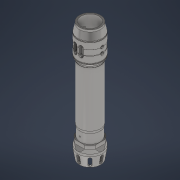
# Autodesk Inventor part: TestPiece1
Saved by Autodesk Inventor 2022 (Build 260153000, 153)
## iProperties
Created: 2024-05-07
Part Number: TestPiece1
Material: Generic
Document SubType Name: Modeling
Designer: jo_ki
Density: 1 g/cm^3
Appearance: Steel - Polished
Author: jo_ki
Autodesk Inventor part; units mm, degrees
sketch "Sketch3" plane through (0, 0, 0) normal (0, 0, 1) x (1, 0, 0)
  line L0 (0, 0) -> (18.25, 0)
  line L1 (18.25, 0) -> (18.25, 106.5)
  line L2 (18.25, 106.5) -> (0, 106.5)
  line L3 (0, 106.5) -> (0, 0)
  line L4 (18.25, 4) -> (18.75, 4)
  line L5 (18.75, 4) -> (18.75, 102.5)
  line L6 (18.75, 102.5) -> (18.25, 102.5)
  line L7 (18.25, 102.5) -> (18.25, 4)
  line L8 (0, -94.8) -> (0, 204.8) projected
  line L9 (22, -29.5) -> (22, -33.5)
  line L10 (22, -33.5) -> (19, -52)
  line L11 (19, -52) -> (0, -52)
  line L12 (0, -52) -> (0, 0)
  line L13 (18.25, 0) -> (20.5, -17)
  line L14 (20.5, -17) -> (20.5, -23.5)
  line L15 (20.5, -23.5) -> (22, -29.5)
  line L16 (16, -52) -> (16, 106.5)
  line L17 (-4.4, 0) -> (26.4, 0) construction
  line L18 (18.25, 106.5) -> (20.5, 106.5)
  line L19 (20.5, 106.5) -> (22, 109.5)
  line L20 (22, 109.5) -> (22, 110.5)
  line L21 (22, 110.5) -> (21.5, 110.5)
  line L22 (21.5, 110.5) -> (21.5, 112)
  line L23 (21.5, 112) -> (22, 112)
  line L24 (22, 112) -> (22, 123)
  line L25 (22, 123) -> (21.5, 123.5)
  line L26 (21.5, 123.5) -> (21.5, 132.5)
  line L27 (21.5, 132.5) -> (22, 133)
  line L28 (22, 133) -> (22, 144)
  line L29 (22, 144) -> (21.5, 144)
  line L30 (21.5, 144) -> (21.5, 145.5)
  line L31 (21.5, 145.5) -> (22, 145.5)
  line L32 (22, 145.5) -> (22, 146.5)
  line L33 (22, 146.5) -> (19, 158.5)
  line L34 (19, 158.5) -> (19, 162)
  line L35 (19, 162) -> (0, 162)
  line L36 (16, 106.5) -> (16, 162)
  line L37 (14, 162) -> (14, 152)
  line L38 (14, 152) -> (16, 152)
  line L39 (18, 0) -> (18, -17)
  line L40 (18, -17) -> (20.5, -17)
  point P0 (16.25, 106.5)
  point P1 (16, 0)
  point P2 (20.4357, -17)
  dimension "d3" = 106.5
  dimension "d4" = 36.5
  dimension "d5" = 0.5
  dimension "d6" = 4
  dimension "d7" = 4
  dimension "d29" = 41
  dimension "d30" = 44
  dimension "d32" = 23.5
  dimension "d33" = 29.5
  dimension "d34" = 33.5
  dimension "d35" = 52
  dimension "d36" = 38
  dimension "d42" = 41
  dimension "d43" = 44
  dimension "d44" = 109.5
  dimension "d45" = 110.5
  dimension "d46" = 43
  dimension "d47" = 112
  dimension "d48" = 123
  dimension "d49" = 45
  dimension "d50" = 43
  dimension "d51" = 133
  dimension "d52" = 158.5
  dimension "d53" = 38
  dimension "d54" = 162
  dimension "d60" = 10
  dimension "d61" = 28
  dimension "d81" = 17
  dimension "d83" = 36
  dimension "d97" = 32
  constraints: 78 end point, 17 perpendicular, 15 point on line, 6 parallel, 5 equal length, 3 horizontal, 2 vertical, 1 collinear
  measures "d3" distance between parallel lines of L0 L2
  measures "d4" diameter of L1 L8
  measures "d5" distance between parallel lines of L1 L5
  measures "d6" distance from line of L1.end L6
  measures "d7" distance between parallel lines of L0 L4
  measures "d29" diameter of L13.end L8
  measures "d30" diameter of L9.start L8
  measures "d32" distance from line of L17 L14.end
  measures "d33" distance from line of L9.start L17
  measures "d34" distance from line of L17 L9.end
  measures "d35" distance from line of L17 L10.end
  measures "d36" diameter of L10.end L8
  measures "d42" diameter of L18.end L8
  measures "d43" diameter of L19.end L8
  measures "d44" distance from line of L17 L19.end
  measures "d45" distance from line of L17 L20.end
  measures "d46" diameter of L21.end L8
  measures "d47" distance from line of L17 L23.end
  measures "d48" distance from line of L17 L24.end
  measures "d49" angle of L24 L25
  measures "d50" diameter of L26 L8
  measures "d51" distance from line of L17 L27.end
  measures "d52" distance from line of L17 L33.end
  measures "d53" diameter of L33.end L8
  measures "d54" distance from line of L17 L34.end
  measures "d60" distance of L37.start L37.end
  measures "d61" diameter of L37 L8
  measures "d81" distance between parallel lines of L40 L0
  measures "d83" diameter of L39 L8
  measures "d97" diameter of L36 L8
revolve "Revolution1" add sketch "Sketch3" angle 360 about axis through (0, -10, 0) along (0, 1, 0) contours L0 L16 L2 L1 | L39 L40 L14 L15 L9 L10 L11 L16 L0 | L1 L6 L5 L4 | L36 L35 L34 L33 L32 L31 L30 L29 L28 L27 L26 L25 L24 L23 L22 L21 L20 L19 L18 L2
sketch "Sketch5" plane through (0, 0, 0) normal (0, 0, 1) x (1, 0, 0)
  line L0 (0, -47.5) -> (0, -38) construction
  line L1 (-2.75, -47.5) -> (-2.75, -38)
  line L2 (2.75, -38) -> (2.75, -47.5)
  arc A0 (-2.75, -47.5) -> (2.75, -47.5) centre (0, -47.5) ccw
  arc A1 (2.75, -38) -> (-2.75, -38) centre (0, -38) ccw
  line L3 (-22, -33.5) -> (22, -33.5) projected
  line L4 (-19, -52) -> (19, -52) projected
  line L5 (0, -33.5) -> (0, -52) construction
  point P0 (0, 0)
  point P1 (0, -42.75)
  point P2 (0, -42.75)
  dimension "d15" = 5.5
  dimension "d16" = 15
  constraints: 10 end point, 4 midpoint, 4 point on circle, 4 tangent, 2 centre point, 1 coincident, 1 parallel, 1 vertical
  measures "d15" distance between parallel lines of L1 L2
extrude "Extrusion2" cut sketch "Sketch5" along normal through all
pattern_circular "Circular Pattern1" count 8 over 360 about axis through (0, -10, 0) along (0, 1, 0) of "Extrusion2"
sketch "Sketch6" plane through (0, 0, 0) normal (0, 0, 1) x (1, 0, 0)
  line L0 (20.5, -23.5) -> (18.5, -17)
  line L1 (18.5, -17) -> (20.5, -17)
  line L2 (-20.5, -17) -> (20.5, -17) projected
  line L3 (-20.5, -23.5) -> (20.5, -23.5) projected
  line L4 (20.5, -17) -> (20.5, -23.5)
  line L5 (20.5, -17) -> (20.5, -23.5) projected
  line L6 (-20.5, -23.5) -> (20.5, -23.5) projected
  line L7 (-22, -29.5) -> (22, -29.5) projected
  line L8 (22, -29.5) -> (18.5, -23.5)
  line L9 (18.5, -17) -> (18.5, -23.5)
  line L10 (-20.5, -17) -> (20.5, -17) projected
  line L11 (20.5, -23.5) -> (22, -29.5)
  point P0 (0, 0)
  dimension "d95" = 2
  constraints: 12 end point, 2 point on line, 1 collinear, 1 perpendicular
  measures "d95" distance of L1.end L0.end
extrude "Extrusion3" cut sketch "Sketch6" along normal through all both and the other way through all
pattern_circular "Circular Pattern2" count 4 over 360 about axis through (0, -10, 0) along (0, 1, 0) of "Extrusion3"
sketch "Sketch7" plane through (0, 0, 0) normal (0, 0, 1) x (1, 0, 0)
  line L0 (0, -27.55) -> (0, 165.3) projected
  line L1 (5.125, 134.375) -> (5.125, 121.625) construction
  line L2 (1.75, 134.375) -> (1.75, 121.625)
  line L3 (8.5, 121.625) -> (8.5, 134.375)
  arc A0 (8.5, 134.375) -> (1.75, 134.375) centre (5.125, 134.375) ccw
  arc A1 (1.75, 121.625) -> (8.5, 121.625) centre (5.125, 121.625) ccw
  line L4 (-21.5, 132.5) -> (21.5, 132.5) construction
  line L5 (-21.5, 123.5) -> (21.5, 123.5) construction
  line L6 (-21.5, 132.5) -> (21.5, 132.5) construction
  line L7 (0, 132.5) -> (0, 123.5) construction
  point P0 (0, 0)
  point P1 (5.125, 128)
  point P2 (0, 128)
  dimension "d55" = 6.75
  dimension "d56" = 19.5
  dimension "d57" = 3.5
  constraints: 10 end point, 4 midpoint, 4 point on circle, 4 tangent, 2 centre point, 1 horizontal alignment, 1 parallel, 1 vertical
  measures "d55" distance between parallel lines of L2 L3
  measures "d57" diameter of L2 L0
extrude "Extrusion4" cut sketch "Sketch7" along normal through all both and the other way through all
mirror "Mirror1" about plane through (0, 0, 0) normal (1, 0, 0) of "Extrusion4"
ref_plane "Work Plane1" through (22, 117.5, 0) normal (1, 0, 0) x (0, 1, 0)
sketch "Sketch8" plane through (22, 117.5, 0) normal (1, 0, 0) x (0, 1, 0)
  line L0 (15, 19.7484) -> (6, 19.7484) projected
  line L1 (6, -19.7484) -> (6, -19.7484) projected
  line L2 (6, -19.7484) -> (15, -19.7484) projected
  line L3 (15, 19.7484) -> (15, -19.7484) projected
  line L4 (15, -19.7484) -> (15, 19.7484) projected
  line L5 (15, 0) -> (6, 0)
  line L6 (6, -19.7484) -> (6, -19.7484) projected
  line L7 (10.5, 0) -> (10.5, 5.3964)
  line L8 (44.5, 19) -> (44.5, -19) projected
  point P0 (-117.5, 0)
  point P1 (15.5, 0)
  point P2 (5.5, 0)
  dimension "d64" = 10
  dimension "d76" = 29
  constraints: 4 end point, 3 point on line, 2 midpoint, 1 symmetric about line, 1 vertical
  measures "d64" distance of point (5.5, 0) point (15.5, 0)
  measures "d76" distance from line of L8 point (15.5, 0)
hole "Hole1" at (22, 133, 0) at (22, 123, 0) direction (-1, 0, 0) diameter 2.9 depth 10 counterbore diameter 5.5 counterbore depth 2.9 clearance for "Socket Head Cap Screw DIN EN ISO 4762" size "M2.5" standard "DIN"
ref_plane "Work Plane2" through (-22, 138.5, 0) normal (1, 0, 0) x (0, 1, 0)
sketch "Sketch9" plane through (-22, 138.5, 0) normal (1, 0, 0) x (0, 1, 0)
  line L0 (-6, -19.7484) -> (-15, -19.7484) projected
  line L1 (-15, 19.7484) -> (-15, -19.7484) projected
  line L2 (-15, 19.7484) -> (-6, 19.7484) projected
  line L3 (-6, 19.7484) -> (-6, -19.7484) projected
  line L4 (-6, 19.7484) -> (-6, -19.7484) projected
  line L5 (-6, 0) -> (-15, 0)
  line L6 (-15, 19.7484) -> (-15, -19.7484) projected
  line L7 (-26.5, -6) -> (5.5, -6)
  line L8 (5.5, -6) -> (5.5, 6)
  line L9 (5.5, 6) -> (-26.5, 6)
  line L10 (-26.5, 6) -> (-26.5, -6)
  line L11 (-26.5, -6) -> (5.5, 6) construction
  line L12 (5.5, -6) -> (-26.5, 6) construction
  point P0 (-138.5, 0)
  point P1 (-10.5, 0)
  dimension "d72" = 12
  dimension "d73" = 32
  constraints: 14 end point, 5 midpoint, 2 parallel, 1 horizontal, 1 perpendicular
  measures "d72" distance of L7.end L8.end
  measures "d73" distance between parallel lines of L10 L8
extrude "Extrusion5" cut sketch "Sketch9" along normal blind 10 contours L7 L1 L5 L3 | L3 L9 L8 L7 | L7 L10 L9 L1 | L5 L1 L9 L3
thread "Thread2" size "M33x3.5" class "6H" standard "ANSI Metric M Profile" length 25
ref_plane "Work Plane3" through (0, -8.5, -18) normal (0, 0, 1) x (1, 0, 0)
sketch "Sketch10" plane through (0, -8.5, -18) normal (0, 0, 1) x (1, 0, 0)
  line L0 (-18, 8.5) -> (18, 8.5) projected
  line L1 (-18, -8.5) -> (18, -8.5) projected
  line L2 (-8.8318, -8.5) -> (8.8318, -8.5) projected
  line L3 (0, -8.5) -> (0, 8.5)
  point P0 (0, 0)
  constraints: 3 midpoint, 2 end point
hole "Hole2" at (0, -8.5, -18) direction (0, 0, 1) diameter 2.013 depth 7.6 thread size "M2.5x0.45" class "6H" standard "ISO Metric profile"
pattern_circular "Circular Pattern3" count 2 over 360 about axis through (0, -10, 0) along (0, 1, 0) of "Hole2"
equation "\"d7\" = d6"
equation "\"d50\" = d46"
body "Solid2"
